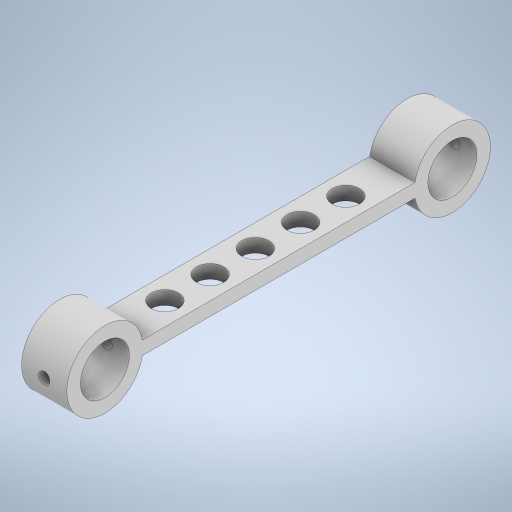
# Autodesk Inventor part: link
Saved by Autodesk Inventor 2024 (Build 280153000, 153)
## iProperties
Created: 2024-07-03
Part Number: link
Material: 일반
Document SubType Name: Modeling
Designer: Gihyeok Na
Density: 1 g/cm^3
Appearance: 기본값
Author: Gihyeok Na
Autodesk Inventor part; units mm, degrees
ref_plane "YZ Plane" through (0, 0, 0) normal (1, 0, 0) x (0, 1, 0)
sketch "스케치1" plane through (0, 0, 0) normal (1, 0, 0) x (0, 1, 0)
  circle A0 centre (0, 0) radius 5.4
  circle A1 centre (0, 0) radius 8.4
  line L0 (34.8065, -38.4) -> (-35.3174, -38.4) construction
  circle A2 centre (0, -76.8) radius 5.4
  circle A3 centre (0, -76.8) radius 8.4
  dimension "d0" = 10.8
  dimension "d1" = 16.8
  dimension "d4" = 38.4
  constraints: 4 centre point, 4 coincident, 3 symmetric about line, 2 end point, 1 horizontal, 2 other
  measures "d0" diameter of A0
  measures "d1" diameter of A1
  measures "d4" distance from line of point (0, 0) L0
extrude "돌출1" add sketch "스케치1" along normal blind 10
ref_plane "작업 평면1" through (0, 0, -8.4) normal (0, 0, 1) x (1, 0, 0)
sketch "스케치2" plane through (0, 0, -8.4) normal (0, 0, 1) x (1, 0, 0)
  line L0 (10, -8.4) -> (10, 8.4) projected
  line L1 (0, -8.4) -> (0, 8.4) projected
  line L2 (0, 8.4) -> (10, 8.4) projected
  line L3 (0, -8.4) -> (10, -8.4) projected
  line L4 (0, -8.4) -> (0, 8.4) projected
  line L5 (10, -1.5) -> (0, -1.5)
  line L6 (0, -1.5) -> (0, 1.5)
  line L7 (0, 1.5) -> (10, 1.5)
  line L8 (10, 1.5) -> (10, -1.5)
  line L9 (10, -1.5) -> (0, 1.5) construction
  line L10 (0, -1.5) -> (10, 1.5) construction
  point P0 (0, 0)
  point P1 (5, 0)
  point P2 (0, -1.5)
  dimension "d6" = 8.4
  dimension "d7" = 3
  dimension "d12" = 10
  constraints: 12 end point, 2 midpoint, 2 parallel, 1 horizontal, 1 perpendicular, 1 point on line
  measures "d6" distance from line of point (5, 0) L2
  measures "d7" distance between parallel lines of L5 L7
  measures "d12" distance of L5.start L5.end
extrude "돌출2" add sketch "스케치2" along normal blind 3 contours L5 L1 L7 L0
extrude "돌출3" add sketch "스케치2" against normal blind 63 contours L5 L1 L7 L0
sketch "스케치4" plane through (0, 1.5, -8.265) normal (0, 1, 0) x (1, 0, 0)
  line L0 (0, 0) -> (0, 60.27) projected
  line L1 (10, 0) -> (0, 0) projected
  line L2 (0, 60.27) -> (10, 60.27) projected
  line L3 (10, 0) -> (10, 60.27) projected
  line L4 (0, 60.27) -> (0, 0) projected
  line L5 (5, -0.4) -> (5, 39.3864) construction
  circle A0 centre (5, 30) radius 3
  circle A1 centre (5, 40) radius 3
  circle A2 centre (5, 50) radius 3
  circle A3 centre (5, 20) radius 3
  circle A4 centre (5, 10) radius 3
  point P0 (0, -8.265)
  dimension "d22" = 6
  dimension "d23" = 30
  dimension "d26" = 10
  dimension "d33" = 10
  constraints: 5 centre point, 3 vertical, 2 end point, 1 point on line, 8 other
  measures "d22" diameter of A0
  measures "d23" distance from line of L1 A0.centre
  measures "d26" distance of A0.centre A1.centre
  measures "d33" distance of A0.centre A3.centre
ref_plane "작업 평면3" through (0, 0, -8.4) normal (0, 0, 1) x (1, 0, 0)
ref_plane "작업 평면4" through (0, 0, -68.4) normal (0, 0, 1) x (1, 0, 0)
extrude "돌출4" cut sketch "스케치4" against normal blind 10 contours A0 | A1 | A2 | A3 | A4
ref_plane "작업 평면6" through (0, 0, -85.2) normal (0, 0, 1) x (1, 0, 0)
ref_plane "작업 평면5" through (0, 0, 8.4) normal (0, 0, 1) x (1, 0, 0)
sketch "스케치5" plane through (0, 0, 8.4) normal (0, 0, 1) x (1, 0, 0)
  line L0 (10, 1.5) -> (0, 1.5) projected
  line L1 (0, 1.5) -> (0, -1.5) projected
  line L2 (0, -1.5) -> (10, -1.5) projected
  line L3 (10, 1.5) -> (10, -1.5) projected
  line L4 (0, 8.4) -> (10, 8.4) projected
  line L5 (0, -8.4) -> (0, 8.4) projected
  line L6 (10, -8.4) -> (10, 8.4) projected
  line L7 (0, -8.4) -> (10, -8.4) projected
  circle A0 centre (5, 0) radius 1.25
  point P0 (0, 0)
  dimension "d40" = 2.5
  dimension "d41" = 5
  dimension "d42" = 8.4
  constraints: 1 centre point
  measures "d40" diameter of A0
  measures "d41" distance from line of L6 A0.centre
  measures "d42" distance from line of A0.centre L4
sketch "스케치6" plane through (0, 0, -85.2) normal (0, 0, 1) x (1, 0, 0)
  circle A0 centre (5, 0) radius 1.25
  line L0 (0, 8.4) -> (10, 8.4) projected
  line L1 (10, -8.4) -> (10, 8.4) projected
  line L2 (10, -1.5) -> (0, -1.5) projected
  line L3 (0, -1.5) -> (0, 1.5) projected
  line L4 (0, 1.5) -> (10, 1.5) projected
  line L5 (10, -1.5) -> (10, 1.5) projected
  line L6 (2, 1.5) -> (2, -1.5) projected
  line L7 (0, -8.4) -> (0, 8.4) projected
  point P0 (0, 0)
  dimension "d46" = 2.5
  dimension "d47" = 8.4
  dimension "d48" = 5
  constraints: 1 centre point
  measures "d46" diameter of A0
  measures "d47" distance from line of L0 A0.centre
  measures "d48" distance from line of L7 A0.centre
extrude "돌출5" cut sketch "스케치6" along normal blind 17 contours A0
extrude "돌출6" cut sketch "스케치5" against normal blind 17 contours A0
